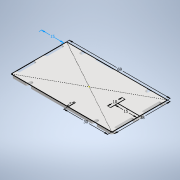
# Autodesk Inventor part: BMS_board
Saved by Autodesk Inventor 2022 (Build 260153000, 153)
## iProperties
Created: 2024-07-26
Part Number: BMS_board
Material: Типовые
Document SubType Name: Modeling
Designer: Капустяник Андрей
Density: 1 g/cm^3
Appearance: По умолчанию
Author: Капустяник Андрей
Autodesk Inventor part; units mm, degrees
ref_plane "YZ Plane" through (0, 0, 0) normal (1, 0, 0) x (0, 1, 0)
ref_plane "XZ Plane" through (0, 0, 0) normal (0, 1, 0) x (-1, 0, 0)
ref_plane "XY Plane" through (0, 0, 0) normal (0, 0, 1) x (1, 0, 0)
sketch "Эскиз1" plane through (0, 0, 0) normal (0, 1, 0) x (-1, 0, 0)
  line L0 (-34.5, 19) -> (34.5, 19)
  line L1 (34.5, 19) -> (34.5, -19)
  line L2 (34.5, -19) -> (-34.5, -19)
  line L3 (-34.5, -19) -> (-34.5, 19)
  line L4 (-34.5, 19) -> (34.5, -19) construction
  line L5 (34.5, 19) -> (-34.5, -19) construction
  line L6 (34.5, -9.5) -> (34.5, 9.5)
  line L7 (36.5, -15.5) -> (32.5, -15.5)
  line L8 (32.5, -15.5) -> (32.5, -3.5)
  line L9 (32.5, -3.5) -> (36.5, -3.5)
  line L10 (36.5, -3.5) -> (36.5, -15.5)
  line L11 (36.5, -15.5) -> (32.5, -3.5) construction
  line L12 (32.5, -15.5) -> (36.5, -3.5) construction
  line L13 (36.5, 3.5) -> (32.5, 3.5)
  line L14 (32.5, 3.5) -> (32.5, 15.5)
  line L15 (32.5, 15.5) -> (36.5, 15.5)
  line L16 (36.5, 15.5) -> (36.5, 3.5)
  line L17 (36.5, 3.5) -> (32.5, 15.5) construction
  line L18 (32.5, 3.5) -> (36.5, 15.5) construction
  line L19 (-34.5, -9.5) -> (-34.5, 9.5)
  line L20 (-32.5, -15.5) -> (-36.5, -15.5)
  line L21 (-36.5, -15.5) -> (-36.5, -3.5)
  line L22 (-36.5, -3.5) -> (-32.5, -3.5)
  line L23 (-32.5, -3.5) -> (-32.5, -15.5)
  line L24 (-32.5, -15.5) -> (-36.5, -3.5) construction
  line L25 (-36.5, -15.5) -> (-32.5, -3.5) construction
  line L26 (-32.5, 3.5) -> (-36.5, 3.5)
  line L27 (-36.5, 3.5) -> (-36.5, 15.5)
  line L28 (-36.5, 15.5) -> (-32.5, 15.5)
  line L29 (-32.5, 15.5) -> (-32.5, 3.5)
  line L30 (-32.5, 3.5) -> (-36.5, 15.5) construction
  line L31 (-36.5, 3.5) -> (-32.5, 15.5) construction
  point P0 (0, 0)
  point P1 (34.5, 0)
  point P2 (-34.5, 0)
  point P3 (-34.5, 15.5)
  point P4 (-34.5, 3.5)
  point P5 (-34.5, -3.5)
  point P6 (-34.5, -15.5)
  point P7 (34.5, -15.5)
  point P8 (34.5, -3.5)
  point P9 (34.5, 3.5)
  point P10 (34.5, 15.5)
  dimension "d0" = 69
  dimension "d1" = 38
  dimension "d4" = 19
  dimension "d5" = 4
  dimension "d6" = 12
  dimension "d7" = 4
  dimension "d8" = 12
  dimension "d9" = 19
  dimension "d10" = 4
  dimension "d11" = 12
  dimension "d12" = 4
  dimension "d13" = 12
  constraints: 64 end point, 14 midpoint, 10 parallel, 5 horizontal, 5 perpendicular, 2 point on line, 1 vertical
  measures "d0" distance of L1.end L2.end
  measures "d1" distance of L0.end L1.end
  measures "d4" distance of L6.start L6.end
  measures "d5" distance of L8.end L9.end
  measures "d6" distance of L7.end L8.end
  measures "d7" distance of L14.end L15.end
  measures "d8" distance of L13.end L14.end
  measures "d9" distance of L19.start L19.end
  measures "d10" distance of L21.end L22.end
  measures "d11" distance of L20.end L21.end
  measures "d12" distance of L27.end L28.end
  measures "d13" distance of L26.end L27.end
extrude "Выдавливание1" add sketch "Эскиз1" along normal blind 2 contours L0 L1 L15 L14 L13 L9 L8 L7 L2 L3 L20 L23 L22 L26 L29 L28
fillet "Сопряжение1" radius 0.5 8 edges at (-32.5, 1, -3.5) (-32.5, 1, -15.5) (-32.5, 1, 3.5) (-32.5, 1, 15.5) (32.5, 1, -15.5) (32.5, 1, -3.5) (32.5, 1, 3.5) (32.5, 1, 15.5)
fillet "Сопряжение2" radius 1 8 edges at (34.5, 1, -3.5) (34.5, 1, 3.5) (34.5, 1, -15.5) (34.5, 1, 15.5) (-34.5, 1, -15.5) (-34.5, 1, -3.5) (-34.5, 1, 3.5) (-34.5, 1, 15.5)
fillet "Сопряжение3" radius 2 4 edges at (-34.5, 1, -19) (-34.5, 1, 19) (34.5, 1, -19) (34.5, 1, 19)
sketch "Эскиз2" plane through (0, 2, 0) normal (0, 1, 0) x (1, 0, 0)
  line L0 (-34.5, -19) -> (34.5, -19)
  line L1 (34.5, -19) -> (34.5, 19)
  line L2 (34.5, 19) -> (-34.5, 19)
  line L3 (-34.5, 19) -> (-34.5, -19)
  line L4 (-34.5, -19) -> (34.5, 19) construction
  line L5 (34.5, -19) -> (-34.5, 19) construction
  line L6 (34.5, -2.5) -> (34.5, 2.5) projected
  line L7 (34.5, 0) -> (19.5, 0)
  line L8 (19.5, 5) -> (19.5, -5)
  line L9 (34.5, -19) -> (4.5, -19)
  line L10 (-32.5, -19) -> (32.5, -19) projected
  line L11 (4.5, -19) -> (4.5, -14)
  point P0 (0, 0)
  dimension "d17" = 69
  dimension "d18" = 38
  dimension "d19" = 15
  dimension "d20" = 10
  dimension "d21" = 30
  dimension "d22" = 5
  constraints: 20 end point, 4 midpoint, 2 horizontal, 2 parallel, 2 perpendicular, 1 point on line, 1 vertical
  measures "d17" distance of L2.end L1.end
  measures "d18" distance of L1.end L0.end
  measures "d19" distance of L7.end L7.start
  measures "d20" distance of L8.start L8.end
  measures "d21" distance of L0.end L9.end
  measures "d22" distance of L9.end L11.end
sketch "Эскиз3" plane through (0, 2, 0) normal (0, 1, 0) x (1, 0, 0)
  arc A0 (32.5, -19) -> (34.5, -17) centre (32.5, -17) ccw projected
  line L0 (34.5, -17) -> (34.5, -16.5) projected
  arc A1 (34.5, -16.5) -> (33.5, -15.5) centre (33.5, -16.5) ccw projected
  line L1 (33.5, -15.5) -> (33, -15.5) projected
  arc A2 (32.5, -15) -> (33, -15.5) centre (33, -15) ccw projected
  line L2 (32.5, -15) -> (32.5, -4) projected
  arc A3 (33, -3.5) -> (32.5, -4) centre (33, -4) ccw projected
  line L3 (33, -3.5) -> (33.5, -3.5) projected
  arc A4 (33.5, -3.5) -> (34.5, -2.5) centre (33.5, -2.5) ccw projected
  line L4 (34.5, -2.5) -> (34.5, 2.5) projected
  arc A5 (34.5, 2.5) -> (33.5, 3.5) centre (33.5, 2.5) ccw projected
  line L5 (33.5, 3.5) -> (33, 3.5) projected
  arc A6 (32.5, 4) -> (33, 3.5) centre (33, 4) ccw projected
  line L6 (32.5, 4) -> (32.5, 15) projected
  arc A7 (33, 15.5) -> (32.5, 15) centre (33, 15) ccw projected
  line L7 (33, 15.5) -> (33.5, 15.5) projected
  arc A8 (33.5, 15.5) -> (34.5, 16.5) centre (33.5, 16.5) ccw projected
  line L8 (34.5, 16.5) -> (34.5, 17) projected
  arc A9 (34.5, 17) -> (32.5, 19) centre (32.5, 17) ccw projected
  line L9 (32.5, 19) -> (-32.5, 19) projected
  arc A10 (-32.5, 19) -> (-34.5, 17) centre (-32.5, 17) ccw projected
  line L10 (-34.5, 17) -> (-34.5, 16.5) projected
  arc A11 (-34.5, 16.5) -> (-33.5, 15.5) centre (-33.5, 16.5) ccw projected
  line L11 (-33.5, 15.5) -> (-33, 15.5) projected
  arc A12 (-32.5, 15) -> (-33, 15.5) centre (-33, 15) ccw projected
  line L12 (-32.5, 15) -> (-32.5, 4) projected
  arc A13 (-33, 3.5) -> (-32.5, 4) centre (-33, 4) ccw projected
  line L13 (-33, 3.5) -> (-33.5, 3.5) projected
  arc A14 (-33.5, 3.5) -> (-34.5, 2.5) centre (-33.5, 2.5) ccw projected
  line L14 (-34.5, 2.5) -> (-34.5, -2.5) projected
  arc A15 (-34.5, -2.5) -> (-33.5, -3.5) centre (-33.5, -2.5) ccw projected
  line L15 (-33.5, -3.5) -> (-33, -3.5) projected
  arc A16 (-32.5, -4) -> (-33, -3.5) centre (-33, -4) ccw projected
  line L16 (-32.5, -4) -> (-32.5, -15) projected
  arc A17 (-33, -15.5) -> (-32.5, -15) centre (-33, -15) ccw projected
  line L17 (-33, -15.5) -> (-33.5, -15.5) projected
  arc A18 (-33.5, -15.5) -> (-34.5, -16.5) centre (-33.5, -16.5) ccw projected
  line L18 (-34.5, -16.5) -> (-34.5, -17) projected
  arc A19 (-34.5, -17) -> (-32.5, -19) centre (-32.5, -17) ccw projected
  line L19 (-32.5, -19) -> (32.5, -19) projected
  circle A20 centre (-22.5, 17.35) radius 1.5 projected
  circle A21 centre (-22.5, -17.35) radius 1.5 projected
  circle A22 centre (-22.5, -17.35) radius 1.1
  circle A23 centre (-22.5, 17.35) radius 1.1
  line L20 (32.5, 19) -> (-32.5, 19) projected
  line L21 (-32.5, -19) -> (32.5, -19) projected
  line L22 (-23.6, 19) -> (-21.4, 19)
  line L23 (-21.4, 19) -> (-21.4, -19)
  line L24 (-21.4, -19) -> (-23.6, -19)
  line L25 (-23.6, -19) -> (-23.6, 19)
  point P0 (0, 0)
  point P1 (-23.6, 16.3302)
  point P2 (-21.4, 16.3302)
  point P3 (-21.4, -19)
  point P4 (-21.4, -16.3302)
  point P5 (-23.6, -16.3302)
  point P6 (-23.6, -17.35)
  point P7 (-21.4, -17.35)
  point P8 (-23.6, 17.35)
  point P9 (-21.4, 17.35)
  dimension "d23" = 2.2
  dimension "d24" = 2.2
  constraints: 8 end point, 2 centre point, 2 coincident, 2 parallel, 2 point on line, 2 tangent, 1 horizontal, 1 perpendicular
  measures "d23" diameter of A22
  measures "d24" diameter of A23
extrude "Выдавливание2" cut sketch "Эскиз3" against normal blind 10 contours L19 L25 A21 L23 | A21 L25 A22 L23 | A22 | L25 L9 L23 A20 | A20 L23 A23 L25 | A23 picked at (-22.5442, -18.7071) picked at (-22.5442, 18.7071)
fillet "Сопряжение4" radius 1 4 edges at (-23.6, 1, 19) (-21.4, 1, 19) (-23.6, 1, -19) (-21.4, 1, -19)
mirror "Зеркальное отражение1" about plane through (0, 0, 0) normal (1, 0, 0) of "Выдавливание2", "Сопряжение4"
sketch "Эскиз4" plane through (0, 2, 0) normal (0, 1, 0) x (1, 0, 0)
  arc A0 (-14, 18.7) -> (-14.3, 19) centre (-14.3, 18.7) ccw projected
  line L0 (-14.3, 19) -> (-26, 19) projected
  arc A1 (-26, 19) -> (-28, 17) centre (-26, 17) ccw projected
  line L1 (-28, 17) -> (-28, -17) projected
  arc A2 (-28, -17) -> (-26, -19) centre (-26, -17) ccw projected
  line L2 (-26, -19) -> (8, -19) projected
  arc A3 (8, -19) -> (10, -17) centre (8, -17) ccw projected
  line L3 (10, -17) -> (10, 17) projected
  arc A4 (10, 17) -> (8, 19) centre (8, 17) ccw projected
  line L4 (8, 19) -> (-1.7, 19) projected
  arc A5 (-1.7, 19) -> (-2, 18.7) centre (-1.7, 18.7) ccw projected
  line L5 (-2, 18.7) -> (-2, 18.3) projected
  arc A6 (-2.3, 18) -> (-2, 18.3) centre (-2.3, 18.3) ccw projected
  line L6 (-2.3, 18) -> (-13.7, 18) projected
  arc A7 (-14, 18.3) -> (-13.7, 18) centre (-13.7, 18.3) ccw projected
  line L7 (-14, 18.3) -> (-14, 18.7) projected
  arc A8 (21.4, 18) -> (20.4, 19) centre (20.4, 18) ccw projected
  line L8 (20.4, 19) -> (-20.4, 19) projected
  arc A9 (-20.4, 19) -> (-21.4, 18) centre (-20.4, 18) ccw projected
  line L9 (-21.4, 18) -> (-21.4, 17.35) projected
  arc A10 (-23.6, 17.35) -> (-21.4, 17.35) centre (-22.5, 17.35) ccw projected
  line L10 (-23.6, 17.35) -> (-23.6, 18) projected
  arc A11 (-23.6, 18) -> (-24.6, 19) centre (-24.6, 18) ccw projected
  line L11 (-24.6, 19) -> (-32.5, 19) projected
  arc A12 (-32.5, 19) -> (-34.5, 17) centre (-32.5, 17) ccw projected
  line L12 (-34.5, 17) -> (-34.5, 16.5) projected
  arc A13 (-34.5, 16.5) -> (-33.5, 15.5) centre (-33.5, 16.5) ccw projected
  line L13 (-33.5, 15.5) -> (-33, 15.5) projected
  arc A14 (-32.5, 15) -> (-33, 15.5) centre (-33, 15) ccw projected
  line L14 (-32.5, 15) -> (-32.5, 4) projected
  arc A15 (-33, 3.5) -> (-32.5, 4) centre (-33, 4) ccw projected
  line L15 (-33, 3.5) -> (-33.5, 3.5) projected
  arc A16 (-33.5, 3.5) -> (-34.5, 2.5) centre (-33.5, 2.5) ccw projected
  line L16 (-34.5, 2.5) -> (-34.5, -2.5) projected
  arc A17 (-34.5, -2.5) -> (-33.5, -3.5) centre (-33.5, -2.5) ccw projected
  line L17 (-33.5, -3.5) -> (-33, -3.5) projected
  arc A18 (-32.5, -4) -> (-33, -3.5) centre (-33, -4) ccw projected
  line L18 (-32.5, -4) -> (-32.5, -15) projected
  arc A19 (-33, -15.5) -> (-32.5, -15) centre (-33, -15) ccw projected
  line L19 (-33, -15.5) -> (-33.5, -15.5) projected
  arc A20 (-33.5, -15.5) -> (-34.5, -16.5) centre (-33.5, -16.5) ccw projected
  line L20 (-34.5, -16.5) -> (-34.5, -17) projected
  arc A21 (-34.5, -17) -> (-32.5, -19) centre (-32.5, -17) ccw projected
  line L21 (-32.5, -19) -> (-24.6, -19) projected
  arc A22 (-24.6, -19) -> (-23.6, -18) centre (-24.6, -18) ccw projected
  line L22 (-23.6, -18) -> (-23.6, -17.35) projected
  arc A23 (-21.4, -17.35) -> (-23.6, -17.35) centre (-22.5, -17.35) ccw projected
  line L23 (-21.4, -17.35) -> (-21.4, -18) projected
  arc A24 (-21.4, -18) -> (-20.4, -19) centre (-20.4, -18) ccw projected
  line L24 (-20.4, -19) -> (20.4, -19) projected
  arc A25 (20.4, -19) -> (21.4, -18) centre (20.4, -18) ccw projected
  line L25 (21.4, -18) -> (21.4, -17.35) projected
  arc A26 (23.6, -17.35) -> (21.4, -17.35) centre (22.5, -17.35) ccw projected
  line L26 (23.6, -17.35) -> (23.6, -18) projected
  arc A27 (23.6, -18) -> (24.6, -19) centre (24.6, -18) ccw projected
  line L27 (24.6, -19) -> (32.5, -19) projected
  arc A28 (32.5, -19) -> (34.5, -17) centre (32.5, -17) ccw projected
  line L28 (34.5, -17) -> (34.5, -16.5) projected
  arc A29 (34.5, -16.5) -> (33.5, -15.5) centre (33.5, -16.5) ccw projected
  line L29 (33.5, -15.5) -> (33, -15.5) projected
  arc A30 (32.5, -15) -> (33, -15.5) centre (33, -15) ccw projected
  line L30 (32.5, -15) -> (32.5, -4) projected
  arc A31 (33, -3.5) -> (32.5, -4) centre (33, -4) ccw projected
  line L31 (33, -3.5) -> (33.5, -3.5) projected
  arc A32 (33.5, -3.5) -> (34.5, -2.5) centre (33.5, -2.5) ccw projected
  line L32 (34.5, -2.5) -> (34.5, 2.5) projected
  arc A33 (34.5, 2.5) -> (33.5, 3.5) centre (33.5, 2.5) ccw projected
  line L33 (33.5, 3.5) -> (33, 3.5) projected
  arc A34 (32.5, 4) -> (33, 3.5) centre (33, 4) ccw projected
  line L34 (32.5, 4) -> (32.5, 15) projected
  arc A35 (33, 15.5) -> (32.5, 15) centre (33, 15) ccw projected
  line L35 (33, 15.5) -> (33.5, 15.5) projected
  arc A36 (33.5, 15.5) -> (34.5, 16.5) centre (33.5, 16.5) ccw projected
  line L36 (34.5, 16.5) -> (34.5, 17) projected
  arc A37 (34.5, 17) -> (32.5, 19) centre (32.5, 17) ccw projected
  line L37 (32.5, 19) -> (24.6, 19) projected
  arc A38 (24.6, 19) -> (23.6, 18) centre (24.6, 18) ccw projected
  line L38 (23.6, 18) -> (23.6, 17.35) projected
  arc A39 (21.4, 17.35) -> (23.6, 17.35) centre (22.5, 17.35) ccw projected
  line L39 (21.4, 17.35) -> (21.4, 18) projected
  point P0 (0, 0)
extrude "Выдавливание3" cut sketch "Эскиз4" against normal blind 10 contours A0 L8 A5 L5 A6 L6 A7 L7
